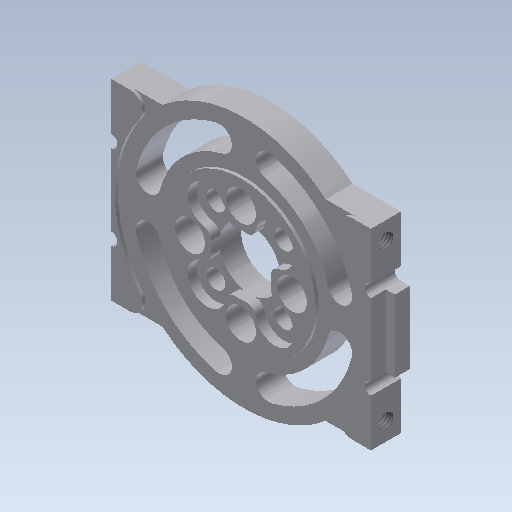
# Autodesk Inventor part: 肩_メインフレーム_1_1
Saved by Autodesk Inventor 2020 (Build 240168000, 168)
## iProperties
Created: 2016-05-05
Part Number: 肩_メインフレーム_1_1
Material: アルミニウム 2014-T4
Document SubType Name: Modeling
Designer: hiroaki
Density: 2.8 g/cm^3
Appearance: サテン
Mass: 13.4242 g
Surface Area: 46.6516 cm^2
Volume: 4.79434 cm^3
Category: 肩
d0: 1.000 ul
d0_1: 10.100 mm
d1: 8.500 mm
d2: 2.700 mm
d3: 5.000 mm
d4: 45.00 deg
d5: 3.100 mm
d6: 5.500 mm
d7: 4.000 ul
d11: 24.900 mm
d12: 42.000 mm
d13: 6.500 mm
d14: 2.100 mm
d15: 4.000 ul
d9: 360.00 deg
d17: 360.00 deg
d19: 24.250 mm
d8: 43.300 mm
d10: 0.000 mm
d16: 1.500 mm
d18: 1.050 mm
d20: 32.000 mm
d21: 10.000 mm
d22: 3.100 mm
d23: 7.000 mm
d24: 5.000 mm
d25: 0.00 deg
d26: 7.000 mm
d28: 2.500 mm
d32: 2.500 mm
d34: 42.100 mm
d35: 0.500 mm
d36: 0.00 deg
d37: 24.900 mm
d38: 5.600 mm
d48: 1.500 mm
d49: 0.00 deg
d50: 2.500 mm
d51: 2.000 mm
d52: 2.000 mm
d53: 2.000 mm
d54: 4.000 ul
d56: 360.00 deg
d58: 5.000 mm
d59: 0.00 deg
d60: 2.100 mm
Author: hiroaki
Autodesk Inventor part; units mm, degrees
ref_plane "YZ Plane" through (0, 0, 0) normal (1, 0, 0) x (0, 1, 0)
ref_plane "XZ Plane" through (0, 0, 0) normal (0, 1, 0) x (-1, 0, 0)
ref_plane "XY Plane" through (0, 0, 0) normal (0, 0, 1) x (1, 0, 0)
derived "付け根ロール_基礎.ipt"
sketch "スケッチ1" plane through (0, 0, 0) normal (0, 0, 1) x (1, 0, 0)
  circle A0 centre (0, 0) radius 5.05 projected
  circle A1 centre (0, -8.5) radius 1.35 construction
  circle A2 centre (0, -8.5) radius 2.5 projected
  circle A3 centre (-5.6569, -5.6569) radius 1.55 projected
  line L0 (-5.6569, -5.6569) -> (0, 0) construction
  line L1 (0, 0) -> (0, -8.5) construction
  line L2 (-4.835, -8.7241) -> (-7.9022, -7.9022) construction
  line L3 (-7.9022, -7.9022) -> (-8.7241, -4.835) construction
  line L4 (-8.7241, -4.835) -> (-6.4787, -2.5896) construction
  line L5 (-6.4787, -2.5896) -> (-3.4115, -3.4115) construction
  line L6 (-3.4115, -3.4115) -> (-2.5896, -6.4787) construction
  line L7 (-2.5896, -6.4787) -> (-4.835, -8.7241) construction
  circle A4 centre (5.6569, -5.6569) radius 1.55 projected
  line L8 (8.7241, -4.835) -> (7.9022, -7.9022) construction
  line L9 (7.9022, -7.9022) -> (4.835, -8.7241) construction
  line L10 (4.835, -8.7241) -> (2.5896, -6.4787) construction
  line L11 (3.4115, -3.4115) -> (6.4787, -2.5896) construction
  line L12 (2.5896, -6.4787) -> (3.4115, -3.4115) construction
  line L13 (6.4787, -2.5896) -> (8.7241, -4.835) construction
  circle A5 centre (8.5, 0) radius 2.5 projected
  circle A6 centre (8.5, 0) radius 1.35 construction
  circle A7 centre (5.6569, 5.6569) radius 1.55 projected
  line L14 (4.835, 8.7241) -> (7.9022, 7.9022) construction
  line L15 (7.9022, 7.9022) -> (8.7241, 4.835) construction
  line L16 (8.7241, 4.835) -> (6.4787, 2.5896) construction
  line L17 (3.4115, 3.4115) -> (2.5896, 6.4787) construction
  line L18 (6.4787, 2.5896) -> (3.4115, 3.4115) construction
  line L19 (2.5896, 6.4787) -> (4.835, 8.7241) construction
  circle A8 centre (0, 8.5) radius 2.5 projected
  circle A9 centre (0, 8.5) radius 1.35 construction
  circle A10 centre (-5.6569, 5.6569) radius 1.55 projected
  line L20 (-8.7241, 4.835) -> (-7.9022, 7.9022) construction
  line L21 (-7.9022, 7.9022) -> (-4.835, 8.7241) construction
  line L22 (-4.835, 8.7241) -> (-2.5896, 6.4787) construction
  line L23 (-3.4115, 3.4115) -> (-6.4787, 2.5896) construction
  line L24 (-2.5896, 6.4787) -> (-3.4115, 3.4115) construction
  line L25 (-6.4787, 2.5896) -> (-8.7241, 4.835) construction
  circle A11 centre (-8.5, 0) radius 2.5 projected
  circle A12 centre (-8.5, 0) radius 1.35 construction
  circle A13 centre (0, 0) radius 12.45 construction
  circle A14 centre (0, 0) radius 21 construction
  circle A15 centre (0, 24.25) radius 3.25 construction
  circle A16 centre (0, 24.25) radius 1.05 construction
  circle A17 centre (-24.25, 0) radius 1.05 construction
  circle A18 centre (0, -24.25) radius 1.05 construction
  circle A19 centre (24.25, 0) radius 1.05 construction
  line L26 (21.65, 16) -> (21.65, 8.1)
  line L27 (-21.65, 16) -> (-21.65, 8.1)
  line L28 (-21.65, 6) -> (-23.15, 6)
  line L29 (-23.15, 6) -> (-23.15, -6)
  line L30 (-23.15, -6) -> (-21.65, -6)
  line L31 (-21.65, -8.1) -> (-21.65, -16)
  line L32 (21.65, -16) -> (21.65, -8.1)
  line L33 (21.65, 6) -> (23.15, 6)
  line L34 (23.15, 6) -> (23.15, -6)
  line L35 (23.15, -6) -> (21.65, -6)
  line L36 (-21.65, 16) -> (-13.6015, 16)
  line L37 (21.65, 16) -> (13.6015, 16)
  arc A20 (13.6015, 16) -> (-13.6015, 16) centre (0, 0) ccw
  arc A21 (-21.65, 6) -> (-21.65, 8.1) centre (-21.65, 7.05) ccw
  line L38 (8.5, 0) -> (0, 0) construction
  arc A22 (-21.65, -8.1) -> (-21.65, -6) centre (-21.65, -7.05) ccw
  arc A23 (21.65, 8.1) -> (21.65, 6) centre (21.65, 7.05) ccw
  arc A24 (21.65, -6) -> (21.65, -8.1) centre (21.65, -7.05) ccw
  line L39 (-21.65, -16) -> (-13.6015, -16)
  arc A25 (-13.6015, -16) -> (13.6015, -16) centre (0, 0) ccw
  line L40 (21.65, -16) -> (13.6015, -16)
  line L41 (-26.8597, 14.55) -> (-19.9642, 14.55) construction
  line L42 (-19.9642, 14.55) -> (-19.9642, 11.45) construction
  line L43 (-19.9642, 11.45) -> (-26.8597, 11.45) construction
  line L44 (-26.8597, 11.45) -> (-26.8597, 14.55) construction
  line L45 (-26.8597, 13) -> (-19.9642, 13) construction
  line L46 (2.75, 25.8377) -> (2.75, 22.6623) projected
  line L47 (2.75, 22.6623) -> (0, 21.0746) projected
  line L48 (0, 21.0746) -> (-2.75, 22.6623) projected
  line L49 (-2.75, 22.6623) -> (-2.75, 25.8377) projected
  line L50 (-2.75, 25.8377) -> (0, 27.4254) projected
  line L51 (0, 27.4254) -> (2.75, 25.8377) projected
  point P0 (0, 21)
  point P1 (-23.15, 0)
  dimension "d8" = 43.3
  dimension "d10" = 0
  dimension "d16" = 1.5
  dimension "d18" = 1.05
  dimension "d20" = 32
  dimension "d21" = 10
  dimension "d22" = 3.1
  dimension "d23" = 7
  constraints: 41 end point, 13 point on circle, 9 symmetric about line, 8 horizontal, 6 centre point, 5 vertical alignment, 4 horizontal alignment, 4 perpendicular, 3 midpoint, 3 parallel, 2 coincident, 2 tangent, 2 vertical, 1 concentric, 6 other
  measures "d8" distance of L27.start L26.start
  measures "d10" radial gap between concentric circles of A20 A14
  measures "d16" distance between parallel lines of L29 L27
  measures "d18" radius of A21
  measures "d20" distance between parallel lines of L39 L36
  measures "d21" distance between parallel lines of L36 L28
  measures "d22" distance of L41.end L42.end
  measures "d23" distance between parallel lines of L28 L45
extrude "押し出し1" add sketch "スケッチ1" along normal blind 5 contours L26 A23 L33 L34 L35 A24 L32 L40 A25 L39 L31 A22 L30 L29 L28 A21 L27 L36 A20 L37
sketch "スケッチ3" plane through (-21.65, 8.1, 0) normal (-1, 0, 0) x (0, 0, 1)
  line L0 (0, 7.9) -> (5, 7.9) projected
  line L1 (5, -5.6) -> (5, -10.6) construction
  line L2 (5, -8.1) -> (0, -8.1) construction
  line L3 (0, -2.1) -> (5, -2.1) projected
  point P0 (2.5, 4.9)
  point P1 (2.5, 7.9)
  point P2 (2.5, -21.1)
  dimension "d26" = 7
  constraints: 2 end point, 2 midpoint, 1 horizontal, 1 symmetric about line, 1 vertical alignment
  measures "d26" distance from line of L3 point (2.5, 4.9)
hole "穴1" at (-21.65, 13, 2.5) at (-21.65, -13, 2.5) direction (1, 0, 0) diameter 2.459 depth 2.5 thread size "M3x0.5" class "6H" standard "ISO Metric profile"
mirror "ミラー1" about plane through (0, 0, 0) normal (1, 0, 0) of "穴1"
sketch "スケッチ4" plane through (0, 0, 5) normal (0, 0, 1) x (1, 0, 0)
  circle A0 centre (0, 0) radius 5.05 projected
  arc A1 (13.6015, 16) -> (-13.6015, 16) centre (0, 0) ccw projected
  circle A2 centre (0, 0) radius 21.05
  circle A3 centre (0, 0) radius 12.45
  dimension "d34" = 42.1
  dimension "d37" = 24.9
  constraints: 2 centre point, 2 coincident
  measures "d34" diameter of A2
  measures "d37" diameter of A3
extrude "押し出し2" cut sketch "スケッチ4" against normal blind 0.5 contours A2
sketch "スケッチ5" plane through (0, 0, 5) normal (0, 0, 1) x (1, 0, 0)
  circle A0 centre (0, 0) radius 12.45 projected
  circle A1 centre (-5.6569, -5.6569) radius 1.55 projected
  circle A2 centre (-5.6569, 5.6569) radius 1.55 projected
  circle A3 centre (5.6569, 5.6569) radius 1.55 projected
  circle A4 centre (5.6569, -5.6569) radius 1.55 projected
  line L0 (-6.4937, 8.7798) -> (-3.3707, 7.943) construction
  line L1 (-3.3707, 7.943) -> (-2.5339, 4.8201) construction
  line L2 (-2.5339, 4.8201) -> (-4.8201, 2.5339) construction
  line L3 (-4.8201, 2.5339) -> (-7.943, 3.3707) construction
  line L4 (-7.943, 3.3707) -> (-8.7798, 6.4937) construction
  line L5 (-8.7798, 6.4937) -> (-6.4937, 8.7798) construction
  arc A5 (-13.6785, 16) -> (-13.6785, -16) centre (0, 0) ccw projected
  circle A6 centre (0, 0) radius 8 construction
  circle A7 centre (0, 0) radius 5.2 construction
  line L6 (-3.3707, 7.943) -> (-2.5339, 4.8201) construction
  line L7 (-2.5339, 4.8201) -> (-4.8201, 2.5339) construction
  line L8 (-4.8201, 2.5339) -> (-7.943, 3.3707) construction
  line L9 (-7.943, 3.3707) -> (-8.7798, 6.4937) construction
  line L10 (-8.7798, 6.4937) -> (-6.4937, 8.7798) construction
  line L11 (-6.4937, 8.7798) -> (-3.3707, 7.943) construction
  line L12 (-5.6569, 5.6569) -> (0, 0) construction
  line L13 (-5.6569, 5.6569) -> (-2.5339, 4.8201) construction
  circle A8 centre (-5.6569, 5.6569) radius 3.2332
  circle A9 centre (-5.6569, -5.6569) radius 3.2332
  circle A10 centre (5.6569, -5.6569) radius 3.2332
  circle A11 centre (5.6569, 5.6569) radius 3.2332
  point P0 (-7.943, 3.3707)
  point P1 (-4.8201, 2.5339)
  point P2 (-2.5339, 4.8201)
  point P3 (-3.3707, 7.943)
  point P4 (-3.677, 3.677)
  point P5 (-8.7798, -6.4937)
  point P6 (6.4937, -8.7798)
  point P7 (8.7798, 6.4937)
  dimension "d38" = 5.6
  dimension "d63" = 5.6
  dimension "d66" = 360
  constraints: 28 end point, 6 collinear, 4 coincident, 1 centre point, 1 midpoint, 1 point on line, 1 tangent, 41 other
  measures "d38" distance between parallel lines of L3 L0
  measures "d63" distance between parallel lines of L8 L11
extrude "押し出し3" cut sketch "スケッチ5" against normal blind 1.5 contours A8 | A9 | A10 | A11
sketch "スケッチ6" plane through (0, 0, 4.5) normal (0, 0, 1) x (0, -1, 0)
  circle A0 centre (0, 0) radius 12.45 projected
  circle A1 centre (0, 0) radius 21.05 projected
  arc A2 (-2, 18.4419) -> (-18.4419, 2) centre (0, 0) ccw
  arc A3 (-2, 14.3109) -> (-14.3109, 2) centre (0, 0) ccw
  line L0 (-2, 18.4419) -> (-2, 14.3109)
  line L1 (-14.3109, 2) -> (-18.4419, 2)
  line L2 (0, 0) -> (0, 21.05) construction
  line L3 (0, 0) -> (-21.05, 0) construction
  arc A4 (-18.4419, -2) -> (-2, -18.4419) centre (0, 0) ccw
  arc A5 (-14.3109, -2) -> (-2, -14.3109) centre (0, 0) ccw
  line L4 (-18.4419, -2) -> (-14.3109, -2)
  line L5 (-2, -14.3109) -> (-2, -18.4419)
  arc A6 (2, -18.4419) -> (18.4419, -2) centre (0, 0) ccw
  arc A7 (2, -14.3109) -> (14.3109, -2) centre (0, 0) ccw
  line L6 (2, -18.4419) -> (2, -14.3109)
  line L7 (14.3109, -2) -> (18.4419, -2)
  arc A8 (18.4419, 2) -> (2, 18.4419) centre (0, 0) ccw
  arc A9 (14.3109, 2) -> (2, 14.3109) centre (0, 0) ccw
  line L8 (18.4419, 2) -> (14.3109, 2)
  line L9 (2, 14.3109) -> (2, 18.4419)
  dimension "d50" = 2.5
  dimension "d51" = 2
  dimension "d52" = 2
  dimension "d53" = 2
  dimension "d56" = 360
  constraints: 20 end point, 18 point on circle, 8 centre point, 2 coincident, 2 parallel, 1 perpendicular, 1 vertical, 41 other
  measures "d50" radial gap between concentric circles of A2 A1
  measures "d51" distance between parallel lines of L2 L0
  measures "d52" radial gap between concentric circles of A0 A3
  measures "d53" distance between parallel lines of L3 L1
extrude "押し出し4" cut sketch "スケッチ6" against normal blind 5 contours L0 A3 L1 A2 | L4 A5 L5 A4 | L6 A7 L7 A6 | L8 A9 L9 A8
fillet "フィレット1" radius 2.1 20 edges at (18.4419, 2, 2.25) (18.4419, -2, 2.25) (14.3109, -2, 2.25) (14.3109, 2, 2.25) (2, 18.4419, 2.25) (2, 14.3109, 2.25) (-2, 14.3109, 2.25) (-2, 18.4419, 2.25) (-14.3109, 2, 2.25) (-14.3109, -2, 2.25) (-18.4419, -2, 2.25) (-18.4419, 2, 2.25) (2, -14.3109, 2.25) (2, -18.4419, 2.25) (-2, -18.4419, 2.25) (-2, -14.3109, 2.25) (-13.6785, 16, 4.75) (-13.6785, -16, 4.75) (13.6785, -16, 4.75) (13.6785, 16, 4.75)
sketch "スケッチ7" plane through (0, 0, 5) normal (0, 0, 1) x (1, 0, 0)
  line L0 (-21.65, 16) -> (-21.65, 8.1) projected
  line L1 (21.65, 8.1) -> (21.65, 16) projected
  line L2 (-28.4103, 9.745) -> (-21.65, 9.745)
  line L3 (-21.65, 9.745) -> (-21.65, -8.8993)
  line L4 (-21.65, -8.8993) -> (-28.4103, -8.8993)
  line L5 (-28.4103, -8.8993) -> (-28.4103, 9.745)
  line L6 (28.1257, 10.9548) -> (21.65, 10.9548)
  line L7 (21.65, 10.9548) -> (21.65, -9.3262)
  line L8 (21.65, -9.3262) -> (28.1257, -9.3262)
  line L9 (28.1257, -9.3262) -> (28.1257, 10.9548)
  constraints: 16 end point, 4 parallel, 2 collinear, 2 horizontal, 2 perpendicular
extrude "押し出し5" cut sketch "スケッチ7" against normal blind 2.5
fillet "フィレット2" radius 1.5 8 edges at (-4.2328, 2.7542, 4.25) (-2.7542, 4.2328, 4.25) (-4.2328, -2.7542, 4.25) (2.7542, 4.2328, 4.25) (4.2328, 2.7542, 4.25) (4.2328, -2.7542, 4.25) (-2.7542, -4.2328, 4.25) (2.7542, -4.2328, 4.25)
equation "\"d26\" = d23"
equation "\"d63\" = d38"
equation "\"d53\" = d51"
